Autodesk Inventor part; units mm, degrees
(part 2 of 2)
sketch "Sketch32" plane through (0, 1.6, 0) normal (0, 1, 0) x (1, 0, 0)
  line L0 (25.095, 13.775) -> (25.095, -13.775)
  line L1 (39.195, 17.1777) -> (33.095, 15.3735)
  line L2 (33.095, 15.3735) -> (33.095, 16.179)
  line L3 (33.095, 16.179) -> (35.0657, 16.7589)
  line L4 (35.0657, 16.7589) -> (35.0657, 18.4718)
  line L5 (35.0657, 18.4718) -> (33.095, 19.0464)
  line L6 (33.095, 19.0464) -> (33.095, 19.8465)
  line L7 (33.095, 19.8465) -> (39.195, 18.0476)
  line L8 (39.195, 18.0476) -> (39.195, 17.1777)
  line L9 (35.6778, 18.3107) -> (35.6778, 16.9146)
  line L10 (35.6778, 16.9146) -> (38.3251, 17.6019)
  line L11 (38.3251, 17.6019) -> (35.6778, 18.3107)
  spline S0 degree 2 poles (33.8682, 12.5651) (34.8402, 12.2107) (37.5841, 11.2496) knots 0 0 0 1 1 1
  line L12 (37.5841, 11.2496) -> (37.5841, 10.4226)
  line L13 (37.5841, 10.4226) -> (33.095, 12.1732)
  line L14 (33.095, 12.1732) -> (33.095, 13.0055)
  line L15 (33.095, 13.0055) -> (37.5841, 14.7399)
  line L16 (37.5841, 14.7399) -> (37.5841, 13.8807)
  line L17 (37.5841, 13.8807) -> (33.8682, 12.5651)
  spline S1 degree 2 poles (33.3044, 8.3875) (33.6212, 8.86) (34.6791, 9.3165) (36.0108, 9.3165) (37.074, 8.8923) (37.7237, 8.0546) (37.7237, 7.5498) knots 0 0 0 1 2 3 4 5 5 5
  spline S2 degree 2 poles (37.7237, 7.5498) (37.7237, 6.5994) (36.4242, 5.7187) (35.4738, 5.7187) knots 0 0 0 1 2 2 2
  line L18 (35.4738, 5.7187) -> (35.2214, 5.7187)
  line L19 (35.2214, 5.7187) -> (35.2214, 8.5593)
  spline S3 degree 2 poles (35.2214, 8.5593) (34.5341, 8.5379) (33.5675, 7.8935) (33.5675, 7.2491) knots 0 0 0 1 2 2 2
  spline S4 degree 2 poles (33.5675, 7.2491) (33.6051, 6.8195) (34.0347, 6.0517) knots 0 0 0 1 1 1
  line L20 (34.0347, 6.0517) -> (33.5246, 5.8047)
  spline S5 degree 2 poles (33.5246, 5.8047) (32.993, 6.3363) (32.993, 7.2599) knots 0 0 0 1 1 1
  spline S6 degree 2 poles (32.993, 7.2599) (32.993, 7.9203) (33.3044, 8.3875) knots 0 0 0 1 1 1
  spline S7 degree 2 poles (35.7691, 6.4276) (37.1491, 6.5081) (37.1491, 7.3941) knots 0 0 0 1 1 1
  spline S8 degree 2 poles (37.1491, 7.3941) (37.1491, 8.3929) (35.7691, 8.5379) knots 0 0 0 1 1 1
  line L21 (35.7691, 8.5379) -> (35.7691, 6.4276)
  line L22 (35.7638, 3.4259) -> (37.5841, 1.4391)
  line L23 (37.5841, 1.4391) -> (37.5841, 0.494)
  line L24 (37.5841, 0.494) -> (35.7208, 2.4969)
  line L25 (35.7208, 2.4969) -> (33.095, 0.2202)
  line L26 (33.095, 0.2202) -> (33.095, 1.1545)
  line L27 (33.095, 1.1545) -> (35.3771, 3.0285)
  line L28 (35.3771, 3.0285) -> (35.0281, 3.4259)
  line L29 (35.0281, 3.4259) -> (33.095, 3.4259)
  line L30 (33.095, 3.4259) -> (33.095, 4.1723)
  line L31 (33.095, 4.1723) -> (39.4205, 4.1723)
  line L32 (39.4205, 4.1723) -> (39.5011, 3.4259)
  line L33 (39.5011, 3.4259) -> (35.7638, 3.4259)
  spline S9 degree 2 poles (33.8682, -2.5291) (34.8402, -2.8835) (37.5841, -3.8447) knots 0 0 0 1 1 1
  line L34 (37.5841, -3.8447) -> (37.5841, -4.6717)
  line L35 (37.5841, -4.6717) -> (33.095, -2.9211)
  line L36 (33.095, -2.9211) -> (33.095, -2.0888)
  line L37 (33.095, -2.0888) -> (37.5841, -0.3544)
  line L38 (37.5841, -0.3544) -> (37.5841, -1.2136)
  line L39 (37.5841, -1.2136) -> (33.8682, -2.5291)
  line L40 (37.0095, -6.0732) -> (37.5841, -6.0732)
  line L41 (37.5841, -6.0732) -> (37.5841, -8.1029)
  line L42 (37.5841, -8.1029) -> (33.6696, -8.1029)
  line L43 (33.6696, -8.1029) -> (33.6696, -9.3863)
  line L44 (33.6696, -9.3863) -> (33.095, -9.3863)
  line L45 (33.095, -9.3863) -> (33.095, -5.9335)
  line L46 (33.095, -5.9335) -> (33.6696, -5.9335)
  line L47 (33.6696, -5.9335) -> (33.6696, -7.3565)
  line L48 (33.6696, -7.3565) -> (37.0095, -7.3565)
  line L49 (37.0095, -7.3565) -> (37.0095, -6.0732)
  line L50 (38.7654, -7.233) -> (39.1735, -7.233)
  spline S10 degree 2 poles (39.1735, -7.233) (39.3185, -7.233) (39.544, -7.5659) (39.544, -7.8935) (39.3185, -8.2264) (39.1735, -8.2264) knots 0 0 0 1 2 3 4 4 4
  line L51 (39.1735, -8.2264) -> (38.7654, -8.2264)
  spline S11 degree 2 poles (38.7654, -8.2264) (38.6204, -8.2264) (38.3949, -7.8935) (38.3949, -7.5659) (38.6204, -7.233) (38.7654, -7.233) knots 0 0 0 1 2 3 4 4 4
  spline S12 degree 2 poles (35.6456, -13.1236) (35.5006, -13.7035) (34.8777, -14.2405) (33.7071, -14.2405) (32.993, -13.3437) (32.993, -12.6725) knots 0 0 0 1 2 3 4 4 4
  spline S13 degree 2 poles (32.993, -12.6725) (32.993, -12.1893) (33.2346, -11.2764) (33.3957, -11.0616) knots 0 0 0 1 2 2 2
  line L52 (33.3957, -11.0616) -> (33.9327, -11.2442)
  spline S14 degree 2 poles (33.9327, -11.2442) (33.8253, -11.416) (33.6105, -12.1624) (33.6105, -13.0323) (33.9756, -13.5532) (34.5824, -13.5532) (34.9261, -13.2954) (35.0174, -12.9303) knots 0 0 0 1 2 3 4 5 6 6 6
  line L53 (35.0174, -12.9303) -> (35.2053, -12.1678)
  spline S15 degree 2 poles (35.2053, -12.1678) (35.3664, -11.5073) (35.9946, -11.0724) (36.9236, -11.0724) (37.713, -11.8295) (37.7183, -12.5544) knots 0 0 0 1 2 3 4 4 4
  line L54 (37.7183, -12.5544) -> (37.7183, -12.6081)
  spline S16 degree 2 poles (37.7183, -12.6081) (37.7183, -13.4243) (37.4123, -13.9935) knots 0 0 0 1 1 1
  line L55 (37.4123, -13.9935) -> (36.8914, -13.8324)
  spline S17 degree 2 poles (36.8914, -13.8324) (37.1438, -13.2364) (37.1438, -12.6188) knots 0 0 0 1 1 1
  spline S18 degree 2 poles (37.1438, -12.6188) (37.1384, -12.243) (36.7679, -11.7543) (36.2041, -11.7543) (35.9195, -12.0013) (35.8389, -12.345) knots 0 0 0 1 2 3 4 4 4
  line L56 (35.8389, -12.345) -> (35.6456, -13.1236)
  line L57 (37.0095, -17.4784) -> (34.9046, -17.4784)
  spline S19 degree 2 poles (34.9046, -17.4784) (34.5126, -17.4784) (34.0508, -17.5643) (33.7662, -17.8221) (33.6696, -18.2356) (33.6696, -18.5846) knots 0 0 0 1 2 3 4 4 4
  line L58 (33.6696, -18.5846) -> (33.6696, -19.4062)
  line L59 (33.6696, -19.4062) -> (33.095, -19.3686)
  line L60 (33.095, -19.3686) -> (33.095, -18.6168)
  spline S20 degree 2 poles (33.095, -18.6168) (33.095, -17.457) (33.5192, -17.0703) knots 0 0 0 1 1 1
  spline S21 degree 2 poles (33.5192, -17.0703) (33.7984, -16.8233) (34.416, -16.7643) knots 0 0 0 1 1 1
  spline S22 degree 2 poles (34.416, -16.7643) (34.6898, -16.7374) (35.0925, -16.7374) knots 0 0 0 1 1 1
  line L61 (35.0925, -16.7374) -> (37.0095, -16.7374)
  line L62 (37.0095, -16.7374) -> (37.0095, -15.4648)
  line L63 (37.0095, -15.4648) -> (37.5841, -15.5507)
  line L64 (37.5841, -15.5507) -> (37.5841, -16.7374)
  line L65 (37.5841, -16.7374) -> (39.1306, -16.7374)
  line L66 (39.1306, -16.7374) -> (39.3507, -17.4784)
  line L67 (39.3507, -17.4784) -> (37.5841, -17.4784)
  line L68 (37.5841, -17.4784) -> (37.5841, -19.3739)
  line L69 (37.5841, -19.3739) -> (37.0095, -19.3739)
  line L70 (37.0095, -19.3739) -> (37.0095, -17.4784)
  point P0 (0, 0)
  constraints: 2 end point, 2 vertical
extrude "Extrusion32" cut sketch "Sketch32" against normal blind 2
body "Solid2"
